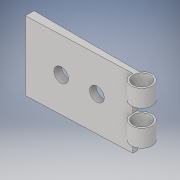
# Autodesk Inventor part: hinge
Saved by Autodesk Inventor 2018 (Build 220112000, 112)
## iProperties
Created: 2019-01-23
Part Number: hinge
Material: Generic
Document SubType Name: Modeling
Designer: s-2513225
Density: 1 g/cm^3
Appearance: Default
Author: s-2513225
Autodesk Inventor part; units mm, degrees
ref_plane "YZ Plane" through (0, 0, 0) normal (1, 0, 0) x (0, 1, 0)
ref_plane "XZ Plane" through (0, 0, 0) normal (0, 1, 0) x (-1, 0, 0)
sketch "Sketch1" plane through (0, 0, 0) normal (0, 0, 1) x (1, 0, 0)
  line L0 (0, 0) -> (38.1, 0)
  line L1 (38.1, 0) -> (38.1, 25.4)
  line L2 (38.1, 25.4) -> (0, 25.4)
  line L3 (0, 25.4) -> (0, 0)
  line L4 (0, 12.7) -> (12.7, 12.7) construction
  line L5 (12.7, 12.7) -> (25.4, 12.7) construction
  circle A0 centre (12.7, 12.7) radius 2.5797
  circle A1 centre (25.4, 12.7) radius 2.5797
  dimension "d0" = 38.1
  dimension "d1" = 25.4
  dimension "d2" = 12.7
  dimension "d3" = 12.7
  dimension "d4" = 5.1594
  dimension "d5" = 5.1594
  constraints: 12 end point, 2 centre point, 2 coincident, 2 horizontal, 2 parallel, 1 midpoint, 1 perpendicular, 1 point on line
  measures "d0" distance of L2.end L1.end
  measures "d1" distance of L1.end L0.end
  measures "d2" distance of L4.start L4.end
  measures "d3" distance of L4.end L5.end
  measures "d4" diameter of A0
  measures "d5" diameter of A1
extrude "Extrusion1" add sketch "Sketch1" along normal blind 3.175
sketch "Sketch2" plane through (0, 25.4, 0) normal (0, 1, 0) x (1, 0, 0)
  circle A0 centre (41.8269, -2.2431) radius 3.175
  arc A1 (38.1, -3.0347) -> (38.7472, 0) centre (41.8269, -2.2431) ccw
  line L0 (0, 0) -> (38.1, 0) projected
  line L1 (38.7472, 0) -> (38.1, 0)
  line L2 (38.1, 0) -> (38.1, -3.175) projected
  line L3 (38.1, 0) -> (38.1, -3.175)
  dimension "d8" = 6.35
  dimension "d9" = 7.62
  constraints: 4 end point, 2 centre point, 2 point on circle, 1 coincident, 1 collinear, 1 horizontal, 1 point on line
  measures "d8" diameter of A0
  measures "d9" diameter of A1
extrude "Extrusion2" add sketch "Sketch2" against normal blind 6.35
ref_plane "Work Plane1" through (0, 12.7, 0) normal (0, -1, 0) x (1, 0, 0)
sketch "Sketch3" plane through (0, 12.7, 0) normal (0, -1, 0) x (1, 0, 0)
  arc A0 (38.7472, 0) -> (38.1, 3.0347) centre (41.8269, 2.2431) ccw projected
  circle A1 centre (41.8269, 2.2431) radius 3.175 projected
  line L0 (38.1, 0) -> (38.7472, 0) projected
  line L1 (38.1, 0) -> (38.1, 3.0347) projected
  line L2 (38.1, 3.0347) -> (38.1, 0)
  point P0 (0, 0)
  constraints: 2 end point, 1 collinear
extrude "Extrusion3" add sketch "Sketch3" along normal blind 6.35
sketch "Sketch4" plane through (0, 25.4, 3.175) normal (0, 1, 0) x (1, 0, 0)
  line L0 (38.1, 0) -> (38.1, 1.3774)
  line L1 (0, 3.175) -> (0, 0) projected
  line L2 (38.1, 1.3774) -> (0, 0)
  line L3 (0, 0) -> (38.1, 0)
  constraints: 6 end point, 1 perpendicular
extrude "Extrusion4" cut sketch "Sketch4" against normal blind 50.8
body "Solid1"
